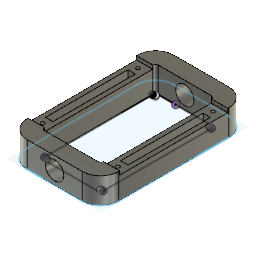
assembly v5 (Autodesk Fusion 360 archive; units mm, degrees)
design "rotor"
Autodesk Fusion 360 part; units mm, degrees
sketch "Sketch1" plane through (0, 0, 0) normal (0, 0, 1) x (1, 0, 0)
  line L0 (0, 0) -> (50, 0)
  line L1 (50, 0) -> (50, 80)
  line L2 (50, 80) -> (0, 80)
  line L3 (0, 80) -> (0, 0)
  line L4 (9, 9) -> (41, 9)
  line L5 (41, 9) -> (41, 71)
  line L6 (41, 71) -> (9, 71)
  line L7 (9, 71) -> (9, 9)
  line L8 (2, 62.5) -> (7, 62.5)
  line L9 (7, 62.5) -> (7, 17.5)
  line L10 (7, 17.5) -> (2, 17.5)
  line L11 (2, 17.5) -> (2, 62.5)
  line L12 (0, 40) -> (2, 40)
  line L13 (25, 71) -> (25, 60)
  line L14 (48, 62.5) -> (43, 62.5)
  line L15 (48, 17.5) -> (48, 62.5)
  line L16 (43, 62.5) -> (43, 17.5)
  line L17 (43, 17.5) -> (48, 17.5)
  dimension "d1" = 50
  dimension "d2" = 80
  dimension "d3" = -9
  dimension "d4" = 45
  dimension "d5" = 90
  dimension "d6" = 2
  dimension "d7" = 5
  constraint horizontal L0
  constraint vertical L1
  constraint horizontal L2
  constraint vertical L3
  constraint coincident L0.start L3.end
  constraint horizontal L8
  constraint vertical L9
  constraint horizontal L10
  constraint vertical L11
  constraint midpoint L3 L12.start
  constraint midpoint L11 L12.end
  constraint midpoint L6 L13.start
  constraint perpendicular L6 L13
  constraint symmetric L8.start L13 L14.start
  constraint symmetric L8.end L13 L14.end
  constraint symmetric L9.end L13 L16.end
  constraint symmetric L10.end L13 L15.start
  measures "d1" distance of L1.end L2.end
  measures "d2" distance of L0.end L1.end
  measures "d4" distance of L8.start L10.end
  measures "d5" angle of L3 L12
  measures "d6" distance of L12.start L12.end
  measures "d7" distance of L8.start L8.end
extrude "Extrude1" add sketch "Sketch1" along normal blind 10
sketch "Sketch2" plane through (0, 0, 0) normal (0, 0, -1) x (1, 0, 0)
  line L0 (2, -17.5) -> (7, -17.5)
  line L1 (7, -17.5) -> (7, -62.5)
  line L2 (7, -62.5) -> (2, -62.5)
  line L3 (2, -62.5) -> (2, -17.5)
  line L4 (43, -17.5) -> (48, -17.5)
  line L5 (48, -17.5) -> (48, -62.5)
  line L6 (48, -62.5) -> (43, -62.5)
  line L7 (43, -62.5) -> (43, -17.5)
  line L8 (9, -71) -> (9, -9)
  line L9 (9, -9) -> (41, -9)
  line L10 (41, -9) -> (41, -71)
  line L11 (41, -71) -> (9, -71)
  line L12 (0, 0) -> (0, -80)
  line L13 (0, -80) -> (50, -80)
  line L14 (50, -80) -> (50, 0)
  line L15 (50, 0) -> (0, 0)
  line L16 (0, 0) -> (50, 0)
  line L17 (50, 0) -> (50, -80)
  line L18 (50, -80) -> (0, -80)
  line L19 (0, -80) -> (0, 0)
  constraint horizontal L16
  constraint vertical L17
  constraint horizontal L18
  constraint vertical L19
  constraint coincident L13.end L14.start
  constraint coincident L12.start L15.end
extrude "Extrude2" add sketch "Sketch2" along normal blind 2 contours L0 L1 L2 L3 | L4 L5 L6 L7 | L12 L13 L14 L15 L16 L17 L18 L19
sketch "Sketch3" plane through (0, 0, 10) normal (0, 0, 1) x (-1, 0, 0)
  line L0 (-7, -17.5) -> (-2, -17.5)
  line L1 (-2, -17.5) -> (-2, -62.5)
  line L2 (-2, -62.5) -> (-7, -62.5)
  line L3 (-7, -62.5) -> (-7, -17.5)
  line L4 (-9, -9) -> (-9, -71)
  line L5 (-9, -71) -> (-41, -71)
  line L6 (-41, -71) -> (-41, -9)
  line L7 (-41, -9) -> (-9, -9)
  line L8 (-48, -17.5) -> (-43, -17.5)
  line L9 (-43, -17.5) -> (-43, -62.5)
  line L10 (-43, -62.5) -> (-48, -62.5)
  line L11 (-48, -62.5) -> (-48, -17.5)
  line L12 (0, -80) -> (0, 0)
  line L13 (0, 0) -> (-50, 0)
  line L14 (-50, 0) -> (-50, -80)
  line L15 (-50, -80) -> (0, -80)
  line L16 (0, -80) -> (-50, -80)
  line L17 (-50, -80) -> (-50, 0)
  line L18 (-50, 0) -> (0, 0)
  line L19 (0, 0) -> (0, -80)
  line L20 (0, -10.5) -> (-50, -10.5)
  line L21 (-50, -10.5) -> (-50, -69.5)
  line L22 (-50, -69.5) -> (0, -69.5)
  line L23 (0, -69.5) -> (0, -10.5)
  line L24 (-4.5, -17.5) -> (-4.5, -10.5)
  line L25 (-4.5, -62.5) -> (-4.5, -69.5)
  line L26 (-45.5, -62.5) -> (-45.5, -69.5)
  line L27 (-45.5, -17.5) -> (-45.5, -10.5)
  circle A0 centre (-4.5, -14) radius 1
  circle A1 centre (-45.5, -14) radius 1
  circle A2 centre (-45.5, -66) radius 1
  circle A3 centre (-4.5, -66) radius 1
  dimension "d12" = 7
  dimension "d13" = 7
  dimension "d14" = 2
  dimension "d15" = 2
  dimension "d16" = 2
  dimension "d17" = 2
  constraint horizontal L16
  constraint vertical L17
  constraint horizontal L18
  constraint vertical L19
  constraint coincident L13.end L14.start
  constraint coincident L12.start L15.end
  constraint horizontal L20
  constraint vertical L21
  constraint horizontal L22
  constraint vertical L23
  constraint coincident L14 L21.end
  constraint coincident L12 L20.start
  constraint midpoint L0 L24.start
  constraint coincident L20 L24.end
  constraint perpendicular L20 L24
  constraint midpoint L2 L25.start
  constraint coincident L22 L25.end
  constraint perpendicular L22 L25
  constraint midpoint L10 L26.start
  constraint coincident L22 L26.end
  constraint perpendicular L22 L26
  constraint midpoint L8 L27.start
  constraint coincident L20 L27.end
  constraint perpendicular L20 L27
  constraint midpoint L24 A0.centre
  constraint midpoint L27 A1.centre
  constraint midpoint L26 A2.centre
  constraint midpoint L25 A3.centre
  measures "d12" distance of L0 L20
  measures "d13" distance of L2 L22
  measures "d14" diameter of A3
  measures "d15" diameter of A2
  measures "d16" diameter of A1
  measures "d17" diameter of A0
extrude "Extrude3" cut sketch "Sketch3" against normal blind 10 contours L24 A0 | L24 A0 | L25 A3 | L25 A3 | L27 A1 | L27 A1 | L26 A2 | L26 A2
extrude "Extrude4" add sketch "Sketch3" along normal blind 2 contours L4 L6 L7 L12 L13 L14 L17 L18 L19 L20 | L4 L5 L6 L12 L14 L15 L16 L17 L19 L22
sketch "Sketch4" plane through (0, 0, 0) normal (0, -1, 0) x (1, 0, 0)
  line L0 (50, -2) -> (50, 12)
  line L1 (50, 12) -> (0, 12)
  line L2 (0, 12) -> (0, -2)
  line L3 (0, -2) -> (50, -2)
  line L4 (25, 12) -> (25, -2)
  circle A0 centre (25, 5) radius 5
  dimension "d22" = 10
  constraint midpoint L1 L4.start
  constraint midpoint L3 L4.end
  constraint midpoint L4 A0.centre
  measures "d22" diameter of A0
extrude "Extrude5" cut sketch "Sketch4" against normal blind 100 contours L4 A0 | L4 A0
sketch "Sketch5" plane through (0, 0, -2) normal (0, 0, -1) x (1, 0, 0)
  line L0 (41, -9) -> (41, -71)
  line L1 (41, -71) -> (9, -71)
  line L2 (9, -71) -> (9, -9)
  line L3 (9, -9) -> (41, -9)
  line L4 (0, -80) -> (50, -80)
  line L5 (50, -80) -> (50, 0)
  line L6 (50, 0) -> (0, 0)
  line L7 (0, 0) -> (0, -80)
  line L8 (10, -80) -> (40, -80)
  line L9 (50, -70) -> (50, -10)
  line L10 (40, 0) -> (10, 0)
  line L11 (0, -10) -> (0, -70)
  line L12 (39.5, -9) -> (10.5, -9)
  line L13 (9, -10.5) -> (9, -69.5)
  line L14 (10.5, -71) -> (39.5, -71)
  line L15 (41, -69.5) -> (41, -10.5)
  arc A0 (10.5, -9) -> (9, -10.5) centre (10.5, -10.5) ccw
  arc A1 (41, -10.5) -> (39.5, -9) centre (39.5, -10.5) ccw
  arc A2 (9, -69.5) -> (10.5, -71) centre (10.5, -69.5) ccw
  arc A3 (39.5, -71) -> (41, -69.5) centre (39.5, -69.5) ccw
  arc A4 (10, 0) -> (0, -10) centre (10, -10) ccw
  arc A5 (50, -10) -> (40, 0) centre (40, -10) ccw
  arc A6 (0, -70) -> (10, -80) centre (10, -70) ccw
  arc A7 (40, -80) -> (50, -70) centre (40, -70) ccw
  point P0 (20, -71)
  point P1 (9, -10.5)
  point P2 (41, -10.5)
  point P3 (41, -69.5)
  point P4 (9, -69.5)
  dimension "d29" = 10
  dimension "d30" = 10
  dimension "d31" = 10
  dimension "d32" = 10
  constraint horizontal L8
  constraint vertical L9
  constraint horizontal L10
  constraint vertical L11
  constraint horizontal L12
  constraint vertical L13
  constraint horizontal L14
  constraint vertical L15
  constraint tangent L12 A0
  constraint tangent L13 A0
  constraint tangent L12 A1
  constraint tangent L15 A1
  constraint tangent L13 A2
  constraint tangent L14 A2
  constraint tangent L14 A3
  constraint tangent L15 A3
  constraint tangent L10 A4
  constraint tangent L11 A4
  constraint tangent L9 A5
  constraint tangent L10 A5
  constraint tangent L8 A6
  constraint tangent L11 A6
  constraint tangent L8 A7
  constraint tangent L9 A7
  constraint coincident L14 P0
  constraint collinear L0 L15
  constraint collinear L3 L12
  constraint collinear L2 L13
  constraint coincident P1 L13.start
  constraint coincident P2 L15.end
  constraint coincident P3 L15.start
  constraint coincident P4 L13.end
  measures "d29" radius of A4
  measures "d30" radius of A5
  measures "d31" radius of A6
  measures "d32" radius of A7
extrude "Extrude6" cut sketch "Sketch5" against normal blind 100 contours L4 L7 A6 | L4 L5 A7 | L6 L7 A4 | L5 L6 A5
extrude "Extrude7" add sketch "Sketch5" against normal up to surface (14 mm away) contours L0 L3 A1 | L0 L1 A3 | L2 L3 A0 | L1 L2 A2
extrude "Extrude8" add 1 faces at (48, 32.5, 3.3333) along direction (-1, 0, 0) blind 0.5
extrude "Extrude9" add 1 faces at (7, 47.5, 3.3333) along direction (-1, 0, 0) blind 0.5
extrude "Extrude10" add 1 faces at (2, 32.5, 3.3333) along direction (1, 0, 0) blind 0.5
extrude "Extrude11" add 1 faces at (43, 47.5, 3.3333) along direction (1, 0, 0) blind 0.5

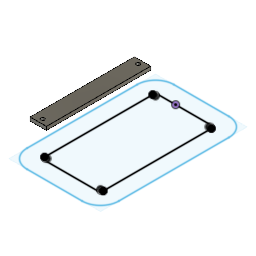
design "rotor_cap"
Autodesk Fusion 360 part; units mm, degrees
sketch "Sketch1" plane through (0, 0, 0) normal (0, 0, 1) x (1, 0, 0)
  line L0 (0, 0) -> (50, 0)
  line L1 (50, 0) -> (50, 80)
  line L2 (50, 80) -> (0, 80)
  line L3 (0, 80) -> (0, 0)
  line L4 (9, 9) -> (41, 9)
  line L5 (41, 9) -> (41, 71)
  line L6 (41, 71) -> (9, 71)
  line L7 (9, 71) -> (9, 9)
  line L8 (2, 62.5) -> (7, 62.5)
  line L9 (7, 62.5) -> (7, 17.5)
  line L10 (7, 17.5) -> (2, 17.5)
  line L11 (2, 17.5) -> (2, 62.5)
  line L12 (0, 40) -> (2, 40)
  line L13 (25, 71) -> (25, 60)
  line L14 (48, 62.5) -> (43, 62.5)
  line L15 (48, 17.5) -> (48, 62.5)
  line L16 (43, 62.5) -> (43, 17.5)
  line L17 (43, 17.5) -> (48, 17.5)
  dimension "d1" = 50
  dimension "d2" = 80
  dimension "d3" = -9
  dimension "d4" = 45
  dimension "d5" = 90
  dimension "d6" = 2
  dimension "d7" = 5
  constraint horizontal L0
  constraint vertical L1
  constraint horizontal L2
  constraint vertical L3
  constraint coincident L0.start L3.end
  constraint horizontal L8
  constraint vertical L9
  constraint horizontal L10
  constraint vertical L11
  constraint midpoint L3 L12.start
  constraint midpoint L11 L12.end
  constraint midpoint L6 L13.start
  constraint perpendicular L6 L13
  constraint symmetric L8.start L13 L14.start
  constraint symmetric L8.end L13 L14.end
  constraint symmetric L9.end L13 L16.end
  constraint symmetric L10.end L13 L15.start
  measures "d1" distance of L1.end L2.end
  measures "d2" distance of L0.end L1.end
  measures "d4" distance of L8.start L10.end
  measures "d5" angle of L3 L12
  measures "d6" distance of L12.start L12.end
  measures "d7" distance of L8.start L8.end
extrude "Extrude1" add sketch "Sketch1" along normal blind 10
sketch "Sketch2" plane through (0, 0, 0) normal (0, 0, -1) x (1, 0, 0)
  line L0 (2, -17.5) -> (7, -17.5)
  line L1 (7, -17.5) -> (7, -62.5)
  line L2 (7, -62.5) -> (2, -62.5)
  line L3 (2, -62.5) -> (2, -17.5)
  line L4 (43, -17.5) -> (48, -17.5)
  line L5 (48, -17.5) -> (48, -62.5)
  line L6 (48, -62.5) -> (43, -62.5)
  line L7 (43, -62.5) -> (43, -17.5)
  line L8 (9, -71) -> (9, -9)
  line L9 (9, -9) -> (41, -9)
  line L10 (41, -9) -> (41, -71)
  line L11 (41, -71) -> (9, -71)
  line L12 (0, 0) -> (0, -80)
  line L13 (0, -80) -> (50, -80)
  line L14 (50, -80) -> (50, 0)
  line L15 (50, 0) -> (0, 0)
  line L16 (0, 0) -> (50, 0)
  line L17 (50, 0) -> (50, -80)
  line L18 (50, -80) -> (0, -80)
  line L19 (0, -80) -> (0, 0)
  constraint horizontal L16
  constraint vertical L17
  constraint horizontal L18
  constraint vertical L19
  constraint coincident L13.end L14.start
  constraint coincident L12.start L15.end
extrude "Extrude2" add sketch "Sketch2" along normal blind 2 contours L0 L1 L2 L3 | L4 L5 L6 L7 | L12 L13 L14 L15 L16 L17 L18 L19
sketch "Sketch3" plane through (0, 0, 10) normal (0, 0, 1) x (-1, 0, 0)
  line L0 (-7, -17.5) -> (-2, -17.5)
  line L1 (-2, -17.5) -> (-2, -62.5)
  line L2 (-2, -62.5) -> (-7, -62.5)
  line L3 (-7, -62.5) -> (-7, -17.5)
  line L4 (-9, -9) -> (-9, -71)
  line L5 (-9, -71) -> (-41, -71)
  line L6 (-41, -71) -> (-41, -9)
  line L7 (-41, -9) -> (-9, -9)
  line L8 (-48, -17.5) -> (-43, -17.5)
  line L9 (-43, -17.5) -> (-43, -62.5)
  line L10 (-43, -62.5) -> (-48, -62.5)
  line L11 (-48, -62.5) -> (-48, -17.5)
  line L12 (0, -80) -> (0, 0)
  line L13 (0, 0) -> (-50, 0)
  line L14 (-50, 0) -> (-50, -80)
  line L15 (-50, -80) -> (0, -80)
  line L16 (0, -80) -> (-50, -80)
  line L17 (-50, -80) -> (-50, 0)
  line L18 (-50, 0) -> (0, 0)
  line L19 (0, 0) -> (0, -80)
  line L20 (0, -10.5) -> (-50, -10.5)
  line L21 (-50, -10.5) -> (-50, -69.5)
  line L22 (-50, -69.5) -> (0, -69.5)
  line L23 (0, -69.5) -> (0, -10.5)
  line L24 (-4.5, -17.5) -> (-4.5, -10.5)
  line L25 (-4.5, -62.5) -> (-4.5, -69.5)
  line L26 (-45.5, -62.5) -> (-45.5, -69.5)
  line L27 (-45.5, -17.5) -> (-45.5, -10.5)
  circle A0 centre (-4.5, -14) radius 1
  circle A1 centre (-45.5, -14) radius 1
  circle A2 centre (-45.5, -66) radius 1
  circle A3 centre (-4.5, -66) radius 1
  dimension "d12" = 7
  dimension "d13" = 7
  dimension "d14" = 2
  dimension "d15" = 2
  dimension "d16" = 2
  dimension "d17" = 2
  constraint horizontal L16
  constraint vertical L17
  constraint horizontal L18
  constraint vertical L19
  constraint coincident L13.end L14.start
  constraint coincident L12.start L15.end
  constraint horizontal L20
  constraint vertical L21
  constraint horizontal L22
  constraint vertical L23
  constraint coincident L14 L21.end
  constraint coincident L12 L20.start
  constraint midpoint L0 L24.start
  constraint coincident L20 L24.end
  constraint perpendicular L20 L24
  constraint midpoint L2 L25.start
  constraint coincident L22 L25.end
  constraint perpendicular L22 L25
  constraint midpoint L10 L26.start
  constraint coincident L22 L26.end
  constraint perpendicular L22 L26
  constraint midpoint L8 L27.start
  constraint coincident L20 L27.end
  constraint perpendicular L20 L27
  constraint midpoint L24 A0.centre
  constraint midpoint L27 A1.centre
  constraint midpoint L26 A2.centre
  constraint midpoint L25 A3.centre
  measures "d12" distance of L0 L20
  measures "d13" distance of L2 L22
  measures "d14" diameter of A3
  measures "d15" diameter of A2
  measures "d16" diameter of A1
  measures "d17" diameter of A0
extrude "Extrude3" cut sketch "Sketch3" against normal blind 10 contours L24 A0 | L24 A0 | L25 A3 | L25 A3 | L27 A1 | L27 A1 | L26 A2 | L26 A2
extrude "Extrude4" add sketch "Sketch3" along normal blind 2 contours L4 L6 L7 L12 L13 L14 L17 L18 L19 L20 | L4 L5 L6 L12 L14 L15 L16 L17 L19 L22
sketch "Sketch4" plane through (0, 0, 0) normal (0, -1, 0) x (1, 0, 0)
  line L0 (50, -2) -> (50, 12)
  line L1 (50, 12) -> (0, 12)
  line L2 (0, 12) -> (0, -2)
  line L3 (0, -2) -> (50, -2)
  line L4 (25, 12) -> (25, -2)
  circle A0 centre (25, 5) radius 5
  dimension "d22" = 10
  constraint midpoint L1 L4.start
  constraint midpoint L3 L4.end
  constraint midpoint L4 A0.centre
  measures "d22" diameter of A0
extrude "Extrude5" cut sketch "Sketch4" against normal blind 100 contours L4 A0 | L4 A0
sketch "Sketch5" plane through (0, 0, -2) normal (0, 0, -1) x (1, 0, 0)
  line L0 (41, -9) -> (41, -71)
  line L1 (41, -71) -> (9, -71)
  line L2 (9, -71) -> (9, -9)
  line L3 (9, -9) -> (41, -9)
  line L4 (0, -80) -> (50, -80)
  line L5 (50, -80) -> (50, 0)
  line L6 (50, 0) -> (0, 0)
  line L7 (0, 0) -> (0, -80)
  line L8 (10, -80) -> (40, -80)
  line L9 (50, -70) -> (50, -10)
  line L10 (40, 0) -> (10, 0)
  line L11 (0, -10) -> (0, -70)
  line L12 (39.5, -9) -> (10.5, -9)
  line L13 (9, -10.5) -> (9, -69.5)
  line L14 (10.5, -71) -> (39.5, -71)
  line L15 (41, -69.5) -> (41, -10.5)
  arc A0 (10.5, -9) -> (9, -10.5) centre (10.5, -10.5) ccw
  arc A1 (41, -10.5) -> (39.5, -9) centre (39.5, -10.5) ccw
  arc A2 (9, -69.5) -> (10.5, -71) centre (10.5, -69.5) ccw
  arc A3 (39.5, -71) -> (41, -69.5) centre (39.5, -69.5) ccw
  arc A4 (10, 0) -> (0, -10) centre (10, -10) ccw
  arc A5 (50, -10) -> (40, 0) centre (40, -10) ccw
  arc A6 (0, -70) -> (10, -80) centre (10, -70) ccw
  arc A7 (40, -80) -> (50, -70) centre (40, -70) ccw
  point P0 (20, -71)
  point P1 (9, -10.5)
  point P2 (41, -10.5)
  point P3 (41, -69.5)
  point P4 (9, -69.5)
  dimension "d29" = 10
  dimension "d30" = 10
  dimension "d31" = 10
  dimension "d32" = 10
  constraint horizontal L8
  constraint vertical L9
  constraint horizontal L10
  constraint vertical L11
  constraint horizontal L12
  constraint vertical L13
  constraint horizontal L14
  constraint vertical L15
  constraint tangent L12 A0
  constraint tangent L13 A0
  constraint tangent L12 A1
  constraint tangent L15 A1
  constraint tangent L13 A2
  constraint tangent L14 A2
  constraint tangent L14 A3
  constraint tangent L15 A3
  constraint tangent L10 A4
  constraint tangent L11 A4
  constraint tangent L9 A5
  constraint tangent L10 A5
  constraint tangent L8 A6
  constraint tangent L11 A6
  constraint tangent L8 A7
  constraint tangent L9 A7
  constraint coincident L14 P0
  constraint collinear L0 L15
  constraint collinear L3 L12
  constraint collinear L2 L13
  constraint coincident P1 L13.start
  constraint coincident P2 L15.end
  constraint coincident P3 L15.start
  constraint coincident P4 L13.end
  measures "d29" radius of A4
  measures "d30" radius of A5
  measures "d31" radius of A6
  measures "d32" radius of A7
extrude "Extrude6" cut sketch "Sketch5" against normal blind 100 contours L4 L7 A6 | L4 L5 A7 | L6 L7 A4 | L5 L6 A5
extrude "Extrude7" add sketch "Sketch5" against normal up to surface (14 mm away) contours L0 L3 A1 | L0 L1 A3 | L2 L3 A0 | L1 L2 A2
sketch "Sketch6" plane through (0, 0, 10) normal (0, 0, 1) x (-1, 0, 0)
  line L0 (-9, -69.5) -> (0, -69.5)
  line L1 (0, -69.5) -> (0, -10.5)
  line L2 (0, -10.5) -> (-9, -10.5)
  line L3 (-9, -10.5) -> (-9, -69.5)
  line L4 (-7, -17.5) -> (-2, -17.5)
  line L5 (-2, -17.5) -> (-2, -62.5)
  line L6 (-2, -62.5) -> (-7, -62.5)
  line L7 (-7, -62.5) -> (-7, -17.5)
  circle A0 centre (-4.5, -66) radius 1
  circle A1 centre (-4.5, -14) radius 1
  line L8 (0, -69.5) -> (-9, -69.5)
  line L9 (-9, -69.5) -> (-9, -10.5)
  line L10 (-9, -10.5) -> (0, -10.5)
  line L11 (0, -10.5) -> (0, -69.5)
  line L12 (12.8472, -89.0472) -> (-65.8375, -89.0472)
  line L13 (-65.8375, -89.0472) -> (-65.8375, 10.3586)
  line L14 (-65.8375, 10.3586) -> (12.8472, 10.3586)
  line L15 (12.8472, 10.3586) -> (12.8472, -89.0472)
  constraint horizontal L8
  constraint vertical L9
  constraint horizontal L10
  constraint vertical L11
  constraint coincident L2.end L3.start
  constraint coincident L0.end L1.start
  constraint horizontal L12
  constraint vertical L13
  constraint horizontal L14
  constraint vertical L15
extrude "Extrude8" cut sketch "Sketch6" against normal blind 100 from surface at 2 contours L12 L13 L14 L15
sketch "Sketch7" plane through (0, 0, 10) normal (0, 0, 1) x (-1, 0, 0)
  line L0 (-9, -69.5) -> (0, -69.5)
  line L1 (0, -69.5) -> (0, -10.5)
  line L2 (0, -10.5) -> (-9, -10.5)
  line L3 (-9, -10.5) -> (-9, -69.5)
  line L4 (-7, -17.5) -> (-2, -17.5)
  line L5 (-2, -17.5) -> (-2, -62.5)
  line L6 (-2, -62.5) -> (-7, -62.5)
  line L7 (-7, -62.5) -> (-7, -17.5)
  circle A0 centre (-4.5, -66) radius 1
  circle A1 centre (-4.5, -14) radius 1
  line L8 (0, -69.5) -> (-9, -69.5)
  line L9 (-9, -69.5) -> (-9, -10.5)
  line L10 (-9, -10.5) -> (0, -10.5)
  line L11 (0, -10.5) -> (0, -69.5)
  constraint horizontal L8
  constraint vertical L9
  constraint horizontal L10
  constraint vertical L11
  constraint coincident L2.end L3.start
  constraint coincident L0.end L1.start
extrude "Extrude9" add sketch "Sketch7" along normal blind 2 contours L0 L1 L2 L3 L8 L9 L10 L11 | L4 L5 L6 L7
sketch "Sketch8" plane through (0, 0, 0) normal (-1, 0, 0) x (0, -1, 0)
  line L0 (-10.5, -2) -> (-10.5, 12)
  line L1 (-10.5, 12) -> (-69.5, 12)
  line L2 (-69.5, 12) -> (-69.5, -2)
  line L3 (-69.5, -2) -> (-10.5, -2)
  line L4 (-69.5, -2) -> (-10.5, -2)
  line L5 (-10.5, -2) -> (-10.5, 10)
  line L6 (-10.5, 10) -> (-69.5, 10)
  line L7 (-69.5, 10) -> (-69.5, -2)
  dimension "d42" = 2
  constraint horizontal L4
  constraint vertical L5
  constraint horizontal L6
  constraint vertical L7
  constraint coincident L0 L5.end
  constraint coincident L2.end L3.start
  measures "d42" distance of L1 L6
extrude "Extrude10" cut sketch "Sketch8" against normal blind 9 contours L0 L2 L3 L4 L5 L6 L7
extrude "Extrude11" cut 1 faces at (3, 10.5, 10.6667) along direction (0, 1, 0) blind 1
extrude "Extrude12" cut 1 faces at (6, 69.5, 11.3333) along direction (0, -1, 0) blind 1

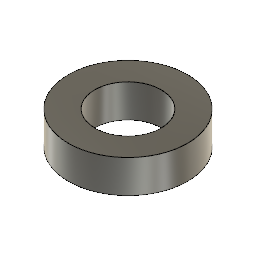
design "washer"
Autodesk Fusion 360 part; units mm, degrees
sketch "Sketch1" plane through (0, 0, 0) normal (0, 0, 1) x (1, 0, 0)
  circle A0 centre (0, 0) radius 5
  circle A1 centre (0, 0) radius 9
  dimension "d1" = 10
  dimension "d2" = 4
  constraint coincident A0.centre A1.centre
  constraint concentric A0 A1
  measures "d1" diameter of A0
  measures "d2" distance of A0 A1
extrude "Extrude1" add sketch "Sketch1" along normal blind 3
extrude "Extrude2" add 1 faces at (7.6145, -0.6955, 3) along direction (0, 0, 1) blind 2

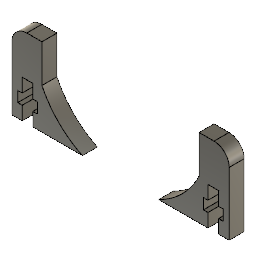
design "stator_stand_for_assem"
Autodesk Fusion 360 part; units mm, degrees
sketch "Sketch1" plane through (0, 0, 0) normal (0, 1, 0) x (1, 0, 0)
  circle A0 centre (0, 0) radius 57.5
  line L0 (-25, -51.7808) -> (25, -51.7808)
  line L1 (51.7808, -25) -> (51.7808, 25)
  line L2 (25, 51.7808) -> (-25, 51.7808)
  line L3 (-51.7808, 25) -> (-51.7808, -25)
  line L4 (-51.7808, 0) -> (-61.7808, 0)
  line L5 (-71.7808, 10) -> (-71.7808, 51.7808)
  line L6 (-71.7808, 51.7808) -> (-25, 51.7808)
  arc A1 (-71.7808, 10) -> (-61.7808, 0) centre (-61.7808, 10) ccw
  line L7 (0, 0) -> (0, 51.7808)
  line L8 (-64.7808, 26.7808) -> (-57.7808, 26.7808)
  line L9 (-57.7808, 26.7808) -> (-57.7808, 51.7808)
  line L10 (-57.7808, 51.7808) -> (-64.7808, 51.7808)
  line L11 (-64.7808, 51.7808) -> (-64.7808, 26.7808)
  line L12 (-67.7808, 35.7808) -> (-54.7808, 35.7808)
  line L13 (-54.7808, 35.7808) -> (-54.7808, 42.7808)
  line L14 (-54.7808, 42.7808) -> (-67.7808, 42.7808)
  line L15 (-67.7808, 42.7808) -> (-67.7808, 35.7808)
  line L16 (-61.2808, 35.7808) -> (-61.2808, 26.7808)
  line L17 (-67.7808, 39.2808) -> (-64.7808, 39.2808)
  line L18 (64.7808, 26.7808) -> (57.7808, 26.7808)
  line L19 (57.7808, 26.7808) -> (57.7808, 51.7808)
  line L20 (64.7808, 51.7808) -> (64.7808, 26.7808)
  line L21 (67.7808, 35.7808) -> (54.7808, 35.7808)
  line L22 (54.7808, 35.7808) -> (54.7808, 42.7808)
  line L23 (67.7808, 42.7808) -> (67.7808, 35.7808)
  line L24 (54.7808, 42.7808) -> (67.7808, 42.7808)
  line L25 (51.7808, 0) -> (61.7808, 0)
  arc A2 (61.7808, 0) -> (71.7808, 10) centre (61.7808, 10) ccw
  line L26 (71.7808, 10) -> (71.7808, 51.7808)
  line L27 (71.7808, 51.7808) -> (25, 51.7808)
  point P0 (-71.7808, 0)
  dimension "d1" = 115
  dimension "d2" = 50
  dimension "d4" = 360
  dimension "d5" = 20
  dimension "d6" = 10
  dimension "d7" = 25
  dimension "d8" = 7
  dimension "d9" = 7
  dimension "d10" = 7
  dimension "d11" = 13
  dimension "d12" = 90
  dimension "d13" = 90
  dimension "d16" = 51.7808
  constraint coincident A0.centre L7.start
  constraint coincident A0 L0.start
  constraint coincident A0 L0.end
  constraint horizontal L0
  constraint midpoint L3 L4.start
  constraint perpendicular L3 L4
  constraint perpendicular L2 L5
  constraint perpendicular L5 L6
  constraint coincident P0 L4
  constraint coincident P0 L5
  constraint tangent L4 A1
  constraint tangent L5 A1
  constraint midpoint L2 L7.end
  constraint horizontal L8
  constraint vertical L9
  constraint horizontal L10
  constraint vertical L11
  constraint coincident L6 L9.end
  constraint horizontal L12
  constraint vertical L13
  constraint horizontal L14
  constraint vertical L15
  constraint midpoint L12 L16.start
  constraint midpoint L8 L16.end
  constraint midpoint L15 L17.start
  constraint midpoint L11 L17.end
  constraint symmetric L2.end L7 L2.start
  constraint symmetric L4.start L7 L25.start
  constraint symmetric L5.end L7 L26.end
  constraint symmetric L4.end L7 L25.end
  constraint symmetric L5.start L7 A2.end
  constraint symmetric A1 L7 A2
  constraint symmetric L7 L8.start L18.start
  constraint symmetric L7 L8.end L18.end
  constraint symmetric L7 L9.end L19.end
  constraint symmetric L7 L10.end L20.start
  constraint symmetric L7 L12.start L21.start
  constraint symmetric L7 L12.end L21.end
  constraint symmetric L7 L13.end L22.end
  constraint symmetric L7 L14.end L23.start
  measures "d1" diameter of A0
  measures "d2" distance of L0.start L0.end
  measures "d5" distance of L4.start P0
  measures "d6" radius of A1
  measures "d7" distance of L8.start L10.end
  measures "d8" distance of L8.start L8.end
  measures "d9" distance of L5 L11
  measures "d10" distance of L12.end L13.end
  measures "d11" distance of L12.start L12.end
  measures "d12" angle of L12 L16
  measures "d13" angle of L15 L17
  measures "d16" distance of A0.centre L7.end
extrude "Extrude1" add sketch "Sketch1" along normal blind 10 contours A0 L1 L25 | A0 L18 L19 L20 L21 L22 L23 L24 L25 A2 L26 L27 | A0 L4 L5 L6 A1 L8 L9 L11 L12 L13 L14 L15 | A0 L3 L4 picked at (55.3786, 2.8629) picked at (-55.3786, 2.8629) makes body 1 at (-63.7808, 0, -12.2603) makes body 2 at (63.7808, 0, -12.2603)

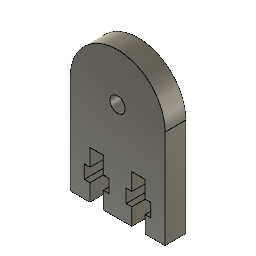
design "rotor_stand"
Autodesk Fusion 360 part; units mm, degrees
sketch "Sketch1" plane through (0, 0, 0) normal (0, 1, 0) x (1, 0, 0)
  circle A0 centre (0, 0) radius 4
  circle A1 centre (0, 0) radius 25
  line L0 (0, 0) -> (-25, 0)
  line L1 (0, 0) -> (25, 0)
  line L2 (-25, 0) -> (25, 0)
  line L3 (25, 0) -> (25, 51.781)
  line L4 (25, 51.781) -> (-25, 51.781)
  line L5 (-25, 51.781) -> (-25, 0)
  line L6 (-14.5, 51.781) -> (-7.5, 51.781)
  line L7 (-7.5, 51.781) -> (-7.5, 26.781)
  line L8 (-7.5, 26.781) -> (-14.5, 26.781)
  line L9 (-14.5, 26.781) -> (-14.5, 51.781)
  line L10 (-17.5, 35.781) -> (-4.5, 35.781)
  line L11 (-4.5, 35.781) -> (-4.5, 42.781)
  line L12 (-4.5, 42.781) -> (-17.5, 42.781)
  line L13 (-17.5, 42.781) -> (-17.5, 35.781)
  line L14 (-11, 35.781) -> (-11, 26.781)
  line L15 (-17.5, 39.281) -> (-14.5, 39.281)
  line L16 (0, 51.781) -> (0, 83.1045)
  line L17 (7.5, 51.781) -> (7.5, 26.781)
  line L18 (7.5, 26.781) -> (14.5, 26.781)
  line L19 (14.5, 26.781) -> (14.5, 51.781)
  line L20 (17.5, 35.781) -> (4.5, 35.781)
  line L21 (17.5, 42.781) -> (17.5, 35.781)
  line L22 (4.5, 42.781) -> (17.5, 42.781)
  line L23 (4.5, 35.781) -> (4.5, 42.781)
  dimension "d1" = 8
  dimension "d2" = 50
  dimension "d3" = 25
  dimension "d4" = 7
  dimension "d5" = 7
  dimension "d6" = 13
  dimension "d7" = 90
  dimension "d8" = 90
  dimension "d9" = 9
  dimension "d10" = 51.781
  constraint coincident A0.centre A1.centre
  constraint coincident A1 L0.end
  constraint horizontal L0
  constraint coincident A1 L1.end
  constraint parallel L0 L1
  constraint horizontal L2
  constraint vertical L3
  constraint horizontal L4
  constraint vertical L5
  constraint horizontal L6
  constraint vertical L7
  constraint horizontal L8
  constraint vertical L9
  constraint coincident L4 L6.start
  constraint horizontal L10
  constraint vertical L11
  constraint horizontal L12
  constraint vertical L13
  constraint midpoint L10 L14.start
  constraint midpoint L8 L14.end
  constraint midpoint L13 L15.start
  constraint midpoint L9 L15.end
  constraint midpoint L4 L16.start
  constraint perpendicular L4 L16
  constraint symmetric L6.start L16 L19.end
  constraint symmetric L6.end L16 L17.start
  constraint symmetric L7.end L16 L17.end
  constraint symmetric L8.end L16 L18.end
  constraint symmetric L10.start L16 L20.start
  constraint symmetric L10.end L16 L20.end
  constraint symmetric L11.end L16 L22.start
  constraint symmetric L12.end L16 L21.start
  measures "d1" diameter of A0
  measures "d2" diameter of A1
  measures "d3" distance of L6.end L7.end
  measures "d4" distance of L7.end L8.end
  measures "d5" distance of L10.start L12.end
  measures "d6" distance of L11 L13
  measures "d7" angle of L8 L14
  measures "d8" angle of L9 L15
  measures "d9" distance of L11 L23
  measures "d10" distance of A0.centre L4
extrude "Extrude1" add sketch "Sketch1" along normal blind 10 contours A0 A1 L0 L1 L2 | A0 A1 L0 L1 L2 | A1 L3 L4 L5 L7 L8 L9 L10 L11 L12 L13 L17 L18 L19 L20 L21 L22 L23
extrude "Extrude2" add 1 faces at (14.2683, 0, -9.6781) along direction (0, -1, 0) blind 1
